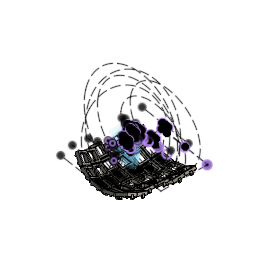
ArcBoard-mk6 v18 (Autodesk Fusion 360 design; units mm, degrees)
part number: mxledbit container
Autodesk Fusion 360 part; units mm, degrees
(part 1 of 5)
ref_plane "WorkPlane2" through (0, 16, 0) normal (0, 1, 0) x (0, 0, 1) in component "IND-Sketch"
sketch "IND-originXY" plane through (0, 0, 0) normal (0, 0, 1) x (1, 0, 0) in component "IND-Sketch"
  line L0 (0, 0) -> (0, 16) construction
  line L1 (0, 16) -> (16, 16) construction
  line L2 (16, 16) -> (16, 0) construction
  line L3 (16, 0) -> (0, 0) construction
  line L4 (0, 16) -> (8, 16) construction
  point P0 (8, 16)
  dimension "d20" = 16
  dimension "d21" = 16
  dimension "d29" = 16
  dimension "d30" = 16
  dimension "d34" = 8
  constraint coincident L0.start L3.end
  constraint vertical L0
  constraint perpendicular L0 L1
  constraint perpendicular L1 L2
  constraint perpendicular L0 L3
  constraint perpendicular L0 L4
  constraint coincident P0 L4.end
  measures "d20" distance of L0.start L0.end
  measures "d21" distance of L0.end L1.end
  measures "d29" distance of L1.end L2.end
  measures "d30" distance of L2.end L0.start
  measures "d34" distance of L0.end P0
sketch "IND-originXZ" plane through (0, 16, 0) normal (0, 1, 0) x (1, 0, 0) in component "IND-Sketch"
  line L0 (0, 0) -> (16, 0) construction
  line L1 (10, 0) -> (10, -10) construction
  line L2 (10, -10) -> (0, -10) construction
  line L3 (0, -10) -> (0, 0) construction
  line L4 (10, -10) -> (5, -10) construction
  line L5 (0, -10) -> (5, -10) construction
  line L6 (0, -10) -> (5, -10) construction
  point P0 (16, 0)
  point P1 (0, -10)
  point P2 (10, -10)
  point P3 (8, 0)
  point P4 (5, -10)
  dimension "d26" = 10
  dimension "d27" = 16
  dimension "d28" = 16
  dimension "d36" = 8
  dimension "d37" = 8
  constraint coincident P0 L1.start
  constraint perpendicular L0 L1
  constraint perpendicular L1 L2
  constraint coincident L0.start L3.end
  constraint coincident P1 L2.end
  constraint coincident P2 L1.end
  constraint midpoint L2 P4
  constraint perpendicular L1 L4
  constraint parallel L4 L6
  measures "d26" distance of L1.start P2
ref_plane "WorkPlane3" through (5, 16, 10) normal (0, 0.866025, -0.5) x (-1, 0, 0) in component "IND-Sketch"
sketch "IND-path" plane through (5, 15.25, 8.701) normal (0, 0.866025, -0.5) x (-1, 0, 0) in component "IND-Sketch"
  line L0 (-5, 1.5) -> (5, 1.5) construction
  line L1 (5, 1.5) -> (-5, 1.5) construction
  circle A0 centre (0, 0) radius 70 construction
  line L2 (0, 0) -> (8, 0) construction
  line L3 (0, 0) -> (-8, 0) construction
  line L4 (0, 0) -> (0, -70) construction
  line L5 (0, -70) -> (6.95, -70) construction
  line L6 (0, -70) -> (-6.95, -70) construction
  point P0 (-5, 1.5)
  point P1 (5, 1.5)
  point P2 (0, -70)
  dimension "d32" = 140
  dimension "d33" = 8
  dimension "d35" = 8
  dimension "d42" = 70
  dimension "d43" = 6.95
  dimension "d44" = 6.95
  dimension "d67" = 90
  constraint coincident P1 L0.end
  constraint coincident P0 L0.start
  constraint coincident A0.centre L2.start
  constraint parallel L1 L2
  constraint parallel L0 L3
  constraint coincident P2 L4.end
  constraint perpendicular L4 L5
  constraint perpendicular L4 L6
  measures "d32" diameter of A0
  measures "d33" distance of A0.centre L2.end
  measures "d35" distance of A0.centre L3.end
  measures "d42" distance of A0.centre P2
  measures "d43" distance of P2 L5.end
  measures "d44" distance of P2 L6.end
  measures "d67" angle of L2 L4
sketch "Sketch1" plane through (5, 15.25, 8.701) normal (0, 0.866025, -0.5) x (-1, 0, 0) in component "wheel"
  circle A0 centre (0, 0) radius 70
  line L0 (0, -70) -> (6.95, -70)
  line L1 (0, -70) -> (-6.95, -70)
  line L2 (0, -70) -> (0, 70) construction
  line L3 (0, 0) -> (70, 0) construction
  circle A1 centre (0, 0) radius 70
  point P0 (0, -70)
  point P1 (0, 1.5)
  dimension "d45" = 140
  dimension "d46" = 70
  dimension "d47" = 140
  constraint coincident P0 L0.start
  constraint perpendicular L0 L2
  constraint coincident A0.centre L3.start
  constraint perpendicular L2 L3
  measures "d45" distance of P0 L2.end
  measures "d46" distance of A0.centre L3.end
  measures "d47" diameter of A1
extrude "Extrude1" add sketch "Sketch1" along normal blind 4 makes body 1 in component "wheel"
ref_plane "WorkPlane1" through (5, -2.4532, -61.9071) normal (0, -0.5, -0.866025) x (1, 0, 0) in component "plug"
sketch "Sketch1 (2)" plane through (5, -4.7032, -60.6081) normal (0, -0.5, -0.866025) x (1, 0, 0) in component "plug"
  line L0 (-70, 13.3745) -> (70, 13.3745)
  line L1 (-70, 13.3745) -> (70, 13.3745)
  line L2 (-70, 17.3745) -> (70, 17.3745)
  line L3 (-70, 17.3745) -> (70, 17.3745)
  line L4 (0, 17.3745) -> (0, 13.3745) construction
  line L5 (0, 17.3745) -> (-6.95, 17.3745) construction
  line L6 (0, 17.3745) -> (6.95, 17.3745) construction
  line L7 (6.95, 17.3745) -> (6.95, 13.3745) construction
  line L8 (-6.95, 17.3745) -> (-6.95, 13.3745) construction
  line L9 (-6.95, 13.3745) -> (6.95, 13.3745) construction
  line L10 (6.95, 13.3745) -> (-6.95, 13.3745)
  line L11 (-6.95, 13.3745) -> (-6.95, 17.3745)
  line L12 (-6.95, 17.3745) -> (6.95, 17.3745)
  line L13 (6.95, 17.3745) -> (6.95, 13.3745)
  point P0 (0, 17.3745)
  dimension "d51" = 6.95
  dimension "d52" = 6.95
  constraint coincident P0 L4.start
  constraint midpoint L1 L4.end
  constraint perpendicular L4 L5
  constraint perpendicular L4 L6
  constraint coincident L1 L7.end
  constraint perpendicular L1 L7
  constraint coincident L0 L8.end
  constraint perpendicular L0 L8
  constraint horizontal L10
  constraint vertical L11
  constraint horizontal L12
  constraint vertical L13
  measures "d51" distance of P0 L5.end
  measures "d52" distance of P0 L6.end
extrude "Extrude1'" add sketch "Sketch1 (2)" along normal blind 4 separate body makes body 2 in component "plug"
sketch "Sketch2" plane through (0, -27.4199, -47.4926) normal (0, 0.5, 0.866025) x (1, 0, 0) in component "plug"
  line L0 (-1.95, 8.8564) -> (11.95, 8.8564)
  line L1 (11.95, 8.8564) -> (11.95, 12.8564)
  line L2 (11.95, 12.8564) -> (-1.95, 12.8564)
  line L3 (-1.95, 12.8564) -> (-1.95, 8.8564)
extrude "Extrude2" add 1 faces at (2.6833, -17.6192, -56.2302) along direction (0, 0.866025, -0.5) blind 4.95 on bodies 2 bodies 2 in component "plug"
extrude "Extrude3" add 1 faces at (7.3167, -20.4167, -53.0755) along direction (0, -0.866025, 0.5) blind 4.95 on bodies 2 bodies 2 in component "plug"
sketch "Sketch1 (3)" plane through (0, 0, 0) normal (0, 0, 1) x (1, 0, 0) in component "main-switchbody (1)"
  line L0 (0, 0) -> (0, 20) construction
  line L1 (0, 20) -> (20, 20) construction
  line L2 (20, 20) -> (20, 0) construction
  line L3 (20, 0) -> (0, 0) construction
  line L4 (0, 0) -> (20, 20) construction
  line L5 (20, 0) -> (0, 20) construction
  line L6 (10, 0) -> (18.9, 0) construction
  line L7 (10, 10) -> (18.9, 10) construction
  line L8 (18.9, 10) -> (18.9, 18.9) construction
  line L9 (18.9, 18.9) -> (1.1, 18.9) construction
  line L10 (1.1, 18.9) -> (1.1, 1.1) construction
  line L11 (1.1, 1.1) -> (18.9, 1.1) construction
  line L12 (18.9, 1.1) -> (18.9, 18.9) construction
  line L13 (10, 10) -> (3.05, 10) construction
  line L14 (3.05, 10) -> (3.05, 16.95) construction
  line L15 (3.05, 16.95) -> (16.95, 16.95) construction
  line L16 (16.95, 16.95) -> (16.95, 3.05) construction
  line L17 (16.95, 3.05) -> (3.05, 3.05) construction
  line L18 (3.05, 3.05) -> (3.05, 16.95) construction
  line L19 (3.05, 3.05) -> (0, 3.05) construction
  line L20 (3.05, 3.05) -> (3.05, 0) construction
  line L21 (16.95, 3.05) -> (20, 3.05) construction
  line L22 (16.95, 16.95) -> (20, 16.95) construction
  line L23 (16.95, 16.95) -> (16.95, 20) construction
  line L24 (3.05, 16.95) -> (3.05, 20) construction
  line L25 (3.05, 16.95) -> (0, 16.95) construction
  line L26 (3.05, 18.9) -> (6.05, 18.9) construction
  line L27 (6.05, 18.9) -> (6.05, 20) construction
  line L28 (16.95, 18.9) -> (13.95, 18.9) construction
  line L29 (13.95, 18.9) -> (13.95, 20) construction
  line L30 (16.95, 3.05) -> (16.95, 0) construction
  line L31 (16.95, 1.1) -> (13.95, 1.1) construction
  line L32 (13.95, 1.1) -> (13.95, 0) construction
  line L33 (3.05, 1.1) -> (6.05, 1.1) construction
  line L34 (6.05, 1.1) -> (6.05, 0) construction
  line L35 (0, 20) -> (20, 20) construction
  line L36 (20, 20) -> (20, 0) construction
  line L37 (20, 0) -> (0, 0) construction
  line L38 (0, 0) -> (0, 20) construction
  line L39 (0, 20) -> (20, 20)
  line L40 (20, 20) -> (20, 0)
  line L41 (20, 0) -> (0, 0)
  line L42 (0, 0) -> (0, 20)
  line L43 (16.95, 3.05) -> (3.05, 3.05)
  line L44 (3.05, 3.05) -> (3.05, 16.95)
  line L45 (3.05, 16.95) -> (16.95, 16.95)
  line L46 (16.95, 16.95) -> (16.95, 3.05)
  line L47 (3.05, 1.1) -> (6.05, 1.1)
  line L48 (6.05, 1.1) -> (6.05, 0)
  line L49 (6.05, 0) -> (3.05, 0)
  line L50 (3.05, 0) -> (3.05, 1.1)
  line L51 (13.95, 1.1) -> (16.95, 1.1)
  line L52 (16.95, 1.1) -> (16.95, 0)
  line L53 (16.95, 0) -> (13.95, 0)
  line L54 (13.95, 0) -> (13.95, 1.1)
  line L55 (13.95, 20) -> (16.95, 20)
  line L56 (16.95, 20) -> (16.95, 18.9)
  line L57 (16.95, 18.9) -> (13.95, 18.9)
  line L58 (13.95, 18.9) -> (13.95, 20)
  line L59 (3.05, 20) -> (6.05, 20)
  line L60 (6.05, 20) -> (6.05, 18.9)
  line L61 (6.05, 18.9) -> (3.05, 18.9)
  line L62 (3.05, 18.9) -> (3.05, 20)
  line L63 (1.1, 10) -> (1.1, 12)
  line L64 (1.1, 10) -> (1.1, 8)
  line L65 (1.1, 8) -> (-1.9, 8)
  line L66 (-1.9, 8) -> (1.1, 8)
  line L67 (1.1, 8) -> (1.1, 12)
  line L68 (1.1, 12) -> (-1.9, 12)
  line L69 (-1.9, 12) -> (-1.9, 8)
  line L70 (3.05, 10) -> (3.05, 7.5) construction
  line L71 (3.05, 7.5) -> (2.55, 7.5) construction
  line L72 (2.55, 7.5) -> (2.55, 12.5) construction
  line L73 (2.55, 12.5) -> (3.05, 12.5085) construction
  line L74 (3.05, 12.5085) -> (3.05, 7.5) construction
  line L75 (2.55, 12.5) -> (16.95, 12.5) construction
  line L76 (16.95, 12.5) -> (17.45, 12.5) construction
  line L77 (17.45, 12.5) -> (17.45, 7.5) construction
  line L78 (17.45, 7.5) -> (16.95, 7.5) construction
  line L79 (16.95, 7.5) -> (16.95, 12.5) construction
  line L80 (17.45, 7.5) -> (16.95, 7.5)
  line L81 (16.95, 7.5) -> (16.95, 12.5)
  line L82 (16.95, 12.5) -> (17.45, 12.5)
  line L83 (17.45, 12.5) -> (17.45, 7.5)
  line L84 (3.05, 7.5) -> (2.55, 7.5)
  line L85 (2.55, 7.5) -> (2.55, 12.5)
  line L86 (2.55, 12.5) -> (3.05, 12.5)
  line L87 (3.05, 12.5) -> (3.05, 7.5)
  dimension "d1_1" = 20
  dimension "d2_1" = 20
  dimension "d3_1" = 8.9
  dimension "d4_1" = 8.9
  dimension "d5_1" = 8.9
  dimension "d6_1" = 17.8
  dimension "d7_1" = 17.8
  dimension "d8_1" = 6.95
  dimension "d9_1" = 6.95
  dimension "d10_1" = 13.9
  dimension "d11_1" = 13.9
  dimension "d12_1" = 13.9
  dimension "d13_1" = 3
  dimension "d14_1" = 3
  dimension "d15_1" = 3
  dimension "d16_1" = 3
  dimension "d21_2" = 3
  dimension "d58_2" = 2.5
  dimension "d59_2" = 0.5
  dimension "d60_2" = 5
  dimension "d61_2" = 0.5
  dimension "d62_2" = 5
  constraint coincident L0.start L3.end
  constraint vertical L0
  constraint perpendicular L0 L1
  constraint perpendicular L1 L2
  constraint perpendicular L0 L3
  constraint midpoint L3 L6.start
  constraint parallel L3 L6
  constraint midpoint L4 L7.start
  constraint parallel L6 L7
  constraint perpendicular L7 L8
  constraint perpendicular L8 L9
  constraint perpendicular L9 L10
  constraint coincident L5 L11.end
  constraint perpendicular L10 L11
  constraint perpendicular L12 L13
  constraint perpendicular L13 L14
  constraint perpendicular L14 L15
  constraint perpendicular L7 L16
  constraint perpendicular L16 L17
  constraint coincident L0 L19.end
  constraint perpendicular L0 L19
  constraint coincident L3 L20.end
  constraint perpendicular L3 L20
  constraint coincident L2 L21.end
  constraint perpendicular L2 L21
  constraint coincident L2 L22.end
  constraint perpendicular L2 L22
  constraint coincident L1 L23.end
  constraint perpendicular L1 L23
  constraint coincident L1 L24.end
  constraint perpendicular L1 L24
  constraint coincident L0 L25.end
  constraint perpendicular L0 L25
  constraint coincident L24 L26.start
  constraint coincident L9 L26.start
  constraint coincident L9 L26.end
  constraint coincident L1 L27.end
  constraint perpendicular L1 L27
  constraint coincident L9 L28.start
  constraint coincident L23 L28.start
  constraint perpendicular L23 L28
  constraint coincident L1 L29.end
  constraint perpendicular L1 L29
  constraint coincident L6 L30.end
  constraint coincident L30 L31.start
  constraint coincident L11 L31.start
  constraint perpendicular L30 L31
  constraint coincident L6 L32.end
  constraint coincident L11 L33.start
  constraint coincident L20 L33.start
  constraint perpendicular L20 L33
  constraint coincident L3 L34.end
  constraint perpendicular L3 L34
  constraint horizontal L35
  constraint vertical L36
  constraint horizontal L37
  constraint vertical L38
  constraint horizontal L39
  constraint vertical L40
  constraint horizontal L41
  constraint vertical L42
  constraint horizontal L43
  constraint vertical L44
  constraint horizontal L45
  constraint vertical L46
  constraint horizontal L47
  constraint vertical L48
  constraint horizontal L49
  constraint vertical L50
  constraint horizontal L51
  constraint vertical L52
  constraint horizontal L53
  constraint vertical L54
  constraint horizontal L55
  constraint vertical L56
  constraint horizontal L57
  constraint vertical L58
  constraint horizontal L59
  constraint vertical L60
  constraint horizontal L61
  constraint vertical L62
  constraint midpoint L10 L63.start
  constraint coincident L10 L63.end
  constraint parallel L10 L63
  constraint coincident L10 L64.end
  constraint perpendicular L0 L65
  constraint horizontal L66
  constraint vertical L67
  constraint horizontal L68
  constraint vertical L69
  constraint perpendicular L13 L70
  constraint perpendicular L70 L71
  constraint perpendicular L71 L72
  constraint coincident L14 L73.end
  constraint perpendicular L71 L74
  constraint coincident L16 L75.end
  constraint perpendicular L16 L75
  constraint perpendicular L16 L76
  constraint perpendicular L76 L77
  constraint coincident L16 L78.end
  constraint perpendicular L16 L78
  constraint horizontal L80
  constraint vertical L81
  constraint horizontal L82
  constraint vertical L83
  constraint horizontal L84
  constraint vertical L85
  constraint horizontal L86
  constraint vertical L87
  measures "d1_1" distance of L0.start L0.end
  measures "d2_1" distance of L0.end L1.end
  measures "d3_1" distance of L6.start L6.end
  measures "d4_1" distance of L7.start L7.end
  measures "d5_1" distance of L7.end L8.end
  measures "d6_1" distance of L8.end L9.end
  measures "d7_1" distance of L9.end L10.end
  measures "d8_1" distance of L7.start L13.end
  measures "d9_1" distance of L13.end L14.end
  measures "d10_1" distance of L14.end L15.end
  measures "d11_1" distance of L15.end L16.end
  measures "d12_1" distance of L16.end L17.end
  measures "d13_1" distance of L26.start L26.end
  measures "d14_1" distance of L28.start L28.end
  measures "d15_1" distance of L31.start L31.end
  measures "d16_1" distance of L33.start L33.end
  measures "d21_2" distance of L64.end L65.end
  measures "d58_2" distance of L13.end L70.end
  measures "d59_2" distance of L70.end L71.end
  measures "d60_2" distance of L71.end L72.end
  measures "d61_2" distance of L75.end L76.end
  measures "d62_2" distance of L76.end L77.end
extrude "Extrude3'" add sketch "Sketch1 (3)" along normal blind 7.5 separate body contours L42 L63 L64 L65 L66 L67 L68 | L42 L65 L66 L68 L69 makes body 3 in component "main-switchbody (1)"
extrude "Extrude2'" add sketch "Sketch1 (3)" along normal blind 4 separate body contours L39 L40 L41 L42 L47 L48 L50 L51 L52 L54 L56 L57 L58 L60 L61 L62 L63 L64 L65 L66 L67 L68 | L42 L63 L64 L65 L66 L67 L68 | L46 L80 L81 L82 L83 | L44 L84 L85 L86 L87 makes body 4 in component "main-switchbody (1)"
extrude "Extrude1''" add sketch "Sketch1 (3)" along normal blind 6 separate body contours L39 L59 L60 L61 L62 | L39 L55 L56 L57 L58 | L41 L47 L48 L49 L50 | L41 L51 L52 L53 L54 makes body 5 at (4.05, 1.1, 2) makes body 6 at (5.05, 20, 4) makes body 7 at (14.95, 1.1, 2) makes body 8 at (14.95, 20, 2) in component "main-switchbody (1)"
extrude "Extrude4" cut sketch "Sketch1 (3)" along normal blind 2 contours L42 L65 L66 L68 L69 bodies 3 in component "main-switchbody (1)"
sketch "Sketch2 (2)" plane through (1.1, 0, 0) normal (1, 0, 0) x (0, 1, 0) in component "main-switchbody (1)"
  line L0 (8, 0) -> (12, 0)
  line L1 (12, 0) -> (12, 7.5)
  line L2 (12, 7.5) -> (8, 7.5)
  line L3 (8, 7.5) -> (8, 0)
  line L4 (8, 7.5) -> (8, 4) construction
  line L5 (8, 4) -> (12, 4) construction
  line L6 (12, 4) -> (12, 7.5) construction
  line L7 (12, 7.5) -> (8, 7.5) construction
  line L8 (8, 7.5) -> (8, 5.75) construction
  line L9 (8, 5.75) -> (12, 5.75) construction
  line L10 (8, 7.5) -> (12, 7.5)
  line L11 (12, 7.5) -> (12, 5.75)
  line L12 (12, 5.75) -> (8, 5.75)
  line L13 (8, 5.75) -> (8, 7.5)
  dimension "d26_2" = 1.75
  constraint coincident L2.end L3.start
  constraint coincident L3 L4.end
  constraint perpendicular L2 L4
  constraint coincident L1 L5.end
  constraint perpendicular L1 L5
  constraint coincident L1.end L2.start
  constraint perpendicular L2 L6
  constraint perpendicular L5 L8
  constraint midpoint L6 L9.end
  constraint horizontal L10
  constraint vertical L11
  constraint horizontal L12
  constraint vertical L13
  measures "d26_2" distance of L2.end L8.end
extrude "Extrude5" add sketch "Sketch2 (2)" along normal blind 1 contours L1 L2 L3 L10 L11 L12 L13 bodies 3 in component "main-switchbody (1)"
extrude "Extrude6" cut 1 faces at (-1.9, 10.6667, 3.8333) along direction (1, 0, 0) blind 1 on bodies 3 bodies 3 in component "main-switchbody (1)"
sketch "Sketch3" plane through (0, 18.9, 0) normal (0, -1, 0) x (1, 0, 0) in component "main-switchbody (1)"
  line L0 (3.05, 0) -> (6.05, 0)
  line L1 (6.05, 0) -> (6.05, 6)
  line L2 (6.05, 6) -> (3.05, 6)
  line L3 (3.05, 6) -> (3.05, 0)
  line L4 (3.05, 6) -> (3.05, 4) construction
  line L5 (6.05, 4) -> (6.05, 6) construction
  line L6 (3.05, 6) -> (3.05, 4.5) construction
  line L7 (6.05, 6) -> (6.05, 4.5) construction
  arc A0 (6.05, 4.5) -> (3.05, 4.5) centre (4.55, 4.5) ccw construction
  arc A1 (6.05, 4.5) -> (3.05, 4.5) centre (4.55, 4.5) ccw
  dimension "d31_2" = 1.5
  dimension "d32_2" = 1.5
  constraint coincident L2.end L3.start
  constraint coincident L3 L4.end
  constraint perpendicular L2 L4
  constraint coincident L1 L5.start
  constraint coincident L1.end L2.start
  constraint perpendicular L2 L5
  constraint perpendicular L2 L6
  constraint perpendicular L2 L7
  constraint tangent L2 A0
  constraint tangent L2 A1
  measures "d31_2" distance of L2.end L6.end
  measures "d32_2" distance of L1.end L7.end
extrude "Extrude7" cut sketch "Sketch3" against normal blind 1.1 contours L2 L3 A1 | L1 L2 A1 bodies 6 in component "main-switchbody (1)"
sketch "Sketch4" plane through (0, 0, 0) normal (0, -1, 0) x (1, 0, 0) in component "main-switchbody (1)"
  line L0 (3.05, 0) -> (6.05, 0)
  line L1 (6.05, 0) -> (6.05, 6)
  line L2 (6.05, 6) -> (3.05, 6)
  line L3 (3.05, 6) -> (3.05, 0)
  line L4 (3.05, 6) -> (3.05, 4.5) construction
  line L5 (6.05, 6) -> (6.05, 4.5) construction
  arc A0 (6.05, 4.5) -> (3.05, 4.5) centre (4.55, 4.5) ccw
  constraint coincident L2.end L3.start
  constraint coincident L3 L4.end
  constraint perpendicular L2 L4
  constraint coincident L1.end L2.start
  constraint coincident L1 L5.end
  constraint perpendicular L2 L5
  constraint tangent L2 A0
extrude "Extrude8" cut sketch "Sketch4" against normal blind 1.1 contours L2 L3 A0 | L1 L2 A0 bodies 5 in component "main-switchbody (1)"
sketch "Sketch5" plane through (0, 0, 0) normal (0, -1, 0) x (1, 0, 0) in component "main-switchbody (1)"
  line L0 (13.95, 0) -> (16.95, 0)
  line L1 (16.95, 0) -> (16.95, 6)
  line L2 (16.95, 6) -> (13.95, 6)
  line L3 (13.95, 6) -> (13.95, 0)
  line L4 (13.95, 6) -> (13.95, 4.5) construction
  line L5 (16.95, 6) -> (16.95, 4.5) construction
  arc A0 (16.95, 4.5) -> (13.95, 4.5) centre (15.45, 4.5) ccw
  constraint coincident L2.end L3.start
  constraint coincident L3 L4.end
  constraint perpendicular L2 L4
  constraint coincident L1.end L2.start
  constraint coincident L1 L5.end
  constraint perpendicular L2 L5
  constraint tangent L2 A0
extrude "Extrude9" cut sketch "Sketch5" against normal blind 1.1 contours L2 L3 A0 | L1 L2 A0 bodies 7 in component "main-switchbody (1)"
sketch "Sketch6" plane through (0, 18.9, 0) normal (0, -1, 0) x (1, 0, 0) in component "main-switchbody (1)"
  line L0 (13.95, 0) -> (16.95, 0)
  line L1 (16.95, 0) -> (16.95, 6)
  line L2 (16.95, 6) -> (13.95, 6)
  line L3 (13.95, 6) -> (13.95, 0)
  line L4 (13.95, 6) -> (13.95, 4.5) construction
  line L5 (16.95, 6) -> (16.95, 4.5) construction
  arc A0 (16.95, 4.5) -> (13.95, 4.5) centre (15.45, 4.5) ccw
  constraint coincident L2.end L3.start
  constraint coincident L3 L4.end
  constraint perpendicular L2 L4
  constraint coincident L1.end L2.start
  constraint coincident L1 L5.end
  constraint perpendicular L2 L5
  constraint tangent L2 A0
extrude "Extrude10" cut sketch "Sketch6" against normal blind 1.1 contours L2 L3 A0 | L1 L2 A0 bodies 8 in component "main-switchbody (1)"
sketch "Sketch7" plane through (0, 0, 4) normal (0, 0, 1) x (-1, 0, 0) in component "main-switchbody (1)"
  line L0 (-3.05, -16.95) -> (-16.95, -16.95)
  line L1 (-16.95, -16.95) -> (-16.95, -3.05)
  line L2 (-16.95, -3.05) -> (-3.05, -3.05)
  line L3 (-3.05, -3.05) -> (-3.05, -16.95)
  line L4 (-6.05, -20) -> (-6.05, -18.9)
  line L5 (-6.05, -18.9) -> (-3.05, -18.9)
  line L6 (-3.05, -18.9) -> (-3.05, -20)
  line L7 (-3.05, -20) -> (0, -20)
  line L8 (0, -20) -> (0, 0)
  line L9 (0, 0) -> (-3.05, 0)
  line L10 (-3.05, 0) -> (-3.05, -1.1)
  line L11 (-3.05, -1.1) -> (-6.05, -1.1)
  line L12 (-6.05, -1.1) -> (-6.05, 0)
  line L13 (-6.05, 0) -> (-13.95, 0)
  line L14 (-13.95, 0) -> (-13.95, -1.1)
  line L15 (-13.95, -1.1) -> (-16.95, -1.1)
  line L16 (-16.95, -1.1) -> (-16.95, 0)
  line L17 (-16.95, 0) -> (-20, 0)
  line L18 (-20, 0) -> (-20, -20)
  line L19 (-20, -20) -> (-16.95, -20)
  line L20 (-16.95, -20) -> (-16.95, -18.9)
  line L21 (-16.95, -18.9) -> (-13.95, -18.9)
  line L22 (-13.95, -18.9) -> (-13.95, -20)
  line L23 (-13.95, -20) -> (-6.05, -20)
  line L24 (-20, -10) -> (-20, -11.5) construction
  line L25 (-20, -10) -> (-20, -8.5) construction
  line L26 (-20, -8.5) -> (-19, -8.5) construction
  line L27 (-19, -8.5) -> (-19, -11.5) construction
  line L28 (-19, -11.5) -> (-20, -11.5) construction
  line L29 (-20, -11.5) -> (-21, -11.5) construction
  line L30 (-21, -11.5) -> (-21, -8.5) construction
  line L31 (-21, -8.5) -> (-20, -8.5) construction
  line L32 (-19, -11.5) -> (-21, -11.5)
  line L33 (-21, -11.5) -> (-21, -8.5)
  line L34 (-21, -8.5) -> (-19, -8.5)
  line L35 (-19, -8.5) -> (-19, -11.5)
  dimension "d41_2" = 1.5
  dimension "d42_2" = 1
  constraint midpoint L18 L24.start
  constraint parallel L18 L24
  constraint coincident L18 L25.end
  constraint parallel L18 L25
  constraint perpendicular L25 L26
  constraint perpendicular L26 L27
  constraint perpendicular L24 L29
  constraint perpendicular L29 L30
  constraint horizontal L32
  constraint vertical L33
  constraint horizontal L34
  constraint vertical L35
  measures "d41_2" distance of L24.start L24.end
  measures "d42_2" distance of L24.end L29.end
extrude "Extrude11" add sketch "Sketch7" along normal blind 3 contours L18 L32 L33 L34 | L18 L32 L34 L35 bodies 4 in component "main-switchbody (1)"
extrude "Extrude12" add 1 faces at (20, 8.5, 6) along direction (0, -1, 0) blind 0.5 on bodies 4 bodies 4 in component "main-switchbody (1)"
extrude "Extrude13" add 1 faces at (20, 11.5, 6) along direction (0, 1, 0) blind 0.5 on bodies 4 bodies 4 in component "main-switchbody (1)"
extrude "Extrude14" add 1 faces at (20.3333, 10.6667, 7) along direction (0, 0, 1) blind 0.75 on bodies 4 bodies 4 in component "main-switchbody (1)"
sketch "Sketch8" plane through (0, 0, 4) normal (0, 0, -1) x (1, 0, 0) in component "main-switchbody (1)"
  line L0 (20, -8) -> (20, -12)
  line L1 (20, -12) -> (21, -12)
  line L2 (21, -12) -> (21, -8)
  line L3 (21, -8) -> (20, -8)
  line L4 (20, -12) -> (20, -8)
  constraint coincident L0.end L1.start
  constraint coincident L0.start L3.end
extrude "Extrude15" add sketch "Sketch8" along normal blind 2 bodies 4 in component "main-switchbody (1)"
sketch "Sketch9" plane through (19, 0, 0) normal (-1, 0, 0) x (0, -1, 0) in component "main-switchbody (1)"
  line L0 (-12, 4) -> (-8, 4)
  line L1 (-8, 4) -> (-8, 7.75)
  line L2 (-8, 7.75) -> (-12, 7.75)
  line L3 (-12, 7.75) -> (-12, 4)
  line L4 (-12, 7.75) -> (-12, 5.75) construction
  line L5 (-12, 5.75) -> (-8, 5.75) construction
  line L6 (-12, 7.75) -> (-8, 7.75)
  line L7 (-8, 7.75) -> (-8, 5.75)
  line L8 (-8, 5.75) -> (-12, 5.75)
  line L9 (-12, 5.75) -> (-12, 7.75)
  dimension "d53_2" = 2
  constraint coincident L2.end L3.start
  constraint perpendicular L2 L4
  constraint coincident L1 L5.end
  constraint perpendicular L1 L5
  constraint horizontal L6
  constraint vertical L7
  constraint horizontal L8
  constraint vertical L9
  measures "d53_2" distance of L2.end L4.end
extrude "Extrude16" add sketch "Sketch9" along normal blind 0.5 contours L1 L2 L3 L6 L7 L8 L9 bodies 4 in component "main-switchbody (1)"
extrude "Extrude17" cut 1 faces at (2.1, 9.3333, 6.9167) along direction (-1, 0, 0) blind 0.3 on bodies 3 bodies 3 in component "main-switchbody (1)"
extrude "Extrude18" cut sketch "Sketch1 (3)" along normal blind 2.7 contours L44 L84 L85 L86 L87 bodies 4 in component "main-switchbody (1)"
extrude "Extrude19" cut sketch "Sketch1 (3)" along normal blind 2.7 contours L46 L80 L81 L82 L83 bodies 4 in component "main-switchbody (1)"
extrude "Extrude20" add sketch "Sketch1 (3)" against normal blind 0.2 contours L39 L40 L41 L42 L47 L48 L50 L51 L52 L54 L56 L57 L58 L60 L61 L62 L63 L64 L65 L66 L67 L68 | L39 L59 L60 L61 L62 | L42 L63 L64 L65 L66 L67 L68 | L39 L55 L56 L57 L58 | L41 L47 L48 L49 L50 | L41 L51 L52 L53 L54 bodies 3 4 5 6 7 8 in component "main-switchbody (1)"
fillet "Fillet1" radius 1 2 edges at (21, 10, 7.75) (-0.9, 10, 7.5) on bodies 3 4 in component "main-switchbody (1)"
extrude "Extrude21" add 1 faces at (2.8833, 9.1667, 2.7) along direction (0, 0, -1) blind 2.9 on bodies 3 bodies 3 in component "main-switchbody (1)"
extrude "Extrude22" add 1 faces at (17.1167, 10.8333, 2.7) along direction (0, 0, -1) blind 2.9 on bodies 3 bodies 3 in component "main-switchbody (1)"
sketch "Sketch10" plane through (0, 0, 4) normal (0, 0, 1) x (-1, 0, 0) in component "main-switchbody (1)"
  line L0 (-3.05, -16.95) -> (-16.95, -16.95)
  line L1 (-16.95, -16.95) -> (-16.95, -3.05)
  line L2 (-16.95, -3.05) -> (-3.05, -3.05)
  line L3 (-3.05, -3.05) -> (-3.05, -16.95)
  line L4 (0, -12) -> (-1.1, -12)
  line L5 (-1.1, -12) -> (-1.1, -8)
  line L6 (-1.1, -8) -> (0, -8)
  line L7 (0, -8) -> (0, 0)
  line L8 (0, 0) -> (-3.05, 0)
  line L9 (-3.05, 0) -> (-3.05, -1.1)
  line L10 (-3.05, -1.1) -> (-6.05, -1.1)
  line L11 (-6.05, -1.1) -> (-6.05, 0)
  line L12 (-6.05, 0) -> (-13.95, 0)
  line L13 (-13.95, 0) -> (-13.95, -1.1)
  line L14 (-13.95, -1.1) -> (-16.95, -1.1)
  line L15 (-16.95, -1.1) -> (-16.95, 0)
  line L16 (-16.95, 0) -> (-20, 0)
  line L17 (-20, 0) -> (-20, -8)
  line L18 (-20, -8) -> (-19, -8)
  line L19 (-19, -8) -> (-19, -12)
  line L20 (-19, -12) -> (-20, -12)
  line L21 (-20, -12) -> (-20, -20)
  line L22 (-20, -20) -> (-16.95, -20)
  line L23 (-16.95, -20) -> (-16.95, -18.9)
  line L24 (-16.95, -18.9) -> (-13.95, -18.9)
  line L25 (-13.95, -18.9) -> (-13.95, -20)
  line L26 (-13.95, -20) -> (-6.05, -20)
  line L27 (-6.05, -20) -> (-6.05, -18.9)
  line L28 (-6.05, -18.9) -> (-3.05, -18.9)
  line L29 (-3.05, -18.9) -> (-3.05, -20)
  line L30 (-3.05, -20) -> (0, -20)
  line L31 (0, -20) -> (0, -12)
  line L32 (-3.05, -10) -> (-3.05, -12.5) construction
  line L33 (-3.05, -12.5) -> (-3.05, -7.5) construction
  line L34 (-3.05, -7.5) -> (-2.55, -7.5) construction
  line L35 (-2.55, -7.5) -> (-3.05, -7.5) construction
  line L36 (-3.05, -7.5) -> (-3.05, -12.5) construction
  line L37 (-3.05, -12.5) -> (-2.55, -12.5) construction
  line L38 (-2.55, -12.5) -> (-2.55, -7.5) construction
  line L39 (-3.05, -12.5) -> (-16.95, -12.5) construction
  line L40 (-16.95, -12.5) -> (-16.95, -7.5) construction
  line L41 (-16.95, -7.5) -> (-17.45, -7.5) construction
  line L42 (-17.45, -7.5) -> (-16.95, -7.5) construction
  line L43 (-16.95, -7.5) -> (-16.95, -12.5) construction
  line L44 (-16.95, -12.5) -> (-17.45, -12.5) construction
  line L45 (-17.45, -12.5) -> (-17.45, -7.5) construction
  line L46 (-16.95, -12.5) -> (-17.45, -12.5)
  line L47 (-17.45, -12.5) -> (-17.45, -7.5)
  line L48 (-17.45, -7.5) -> (-16.95, -7.5)
  line L49 (-16.95, -7.5) -> (-16.95, -12.5)
  line L50 (-2.55, -12.5) -> (-3.05, -12.5)
  line L51 (-3.05, -12.5) -> (-3.05, -7.5)
  line L52 (-3.05, -7.5) -> (-2.55, -7.5)
  line L53 (-2.55, -7.5) -> (-2.55, -12.5)
  dimension "d75_1" = 5
  dimension "d76_1" = 0.5
  dimension "d77_1" = 0.5
  constraint midpoint L3 L32.start
  constraint coincident L3 L32.end
  constraint perpendicular L0 L32
  constraint parallel L3 L33
  constraint perpendicular L33 L34
  constraint horizontal L35
  constraint vertical L36
  constraint horizontal L37
  constraint vertical L38
  constraint coincident L1 L39.end
  constraint perpendicular L1 L39
  constraint coincident L1 L40.end
  constraint perpendicular L39 L40
  constraint perpendicular L40 L41
  constraint horizontal L42
  constraint vertical L43
  constraint horizontal L44
  constraint vertical L45
  constraint horizontal L46
  constraint vertical L47
  constraint horizontal L48
  constraint vertical L49
  constraint horizontal L50
  constraint vertical L51
  constraint horizontal L52
  constraint vertical L53
  measures "d75_1" distance of L32.end L33.end
  measures "d76_1" distance of L33.end L34.end
  measures "d77_1" distance of L40.end L41.end
extrude "Extrude23" cut sketch "Sketch10" against normal blind 2.9 contours L3 L50 L51 L52 L53 | L1 L46 L47 L48 L49 bodies 3 in component "main-switchbody (1)"
extrude "Extrude24" cut 2 faces at (4.8122, 18.9, 5.1079) (15.1626, 18.9, 5.4316) along direction (0, 1, 0) blind 0.25 on bodies 3 bodies 3 in component "main-switchbody (1)"
extrude "Extrude25" cut 2 faces at (4.2822, 1.1, 5.1824) (15.2673, 1.1, 4.9654) along direction (0, -1, 0) blind 0.25 on bodies 3 bodies 3 in component "main-switchbody (1)"
extrude "Extrude26" add 1 faces at (1.0167, 12.3167, -0.2) along direction (0, 0, -1) blind 1 on bodies 3 bodies 3 in component "main-switchbody (1)"
extrude "Extrude27" cut 1 faces at (1.0167, 12.3167, -1.2) along direction (0, 0, 1) blind 0.2 on bodies 3 bodies 3 in component "main-switchbody (1)"
extrude "Extrude28" cut 2 faces at (17.1167, 10.8333, 1.1) (2.8833, 9.1667, 1.1) along direction (0, 0, -1) blind 0.8 on bodies 3 bodies 3 in component "main-switchbody (1)"
extrude "Extrude29" cut 1 faces at (18.8333, 9.3333, 5.75) along direction (0, 0, 1) blind 0.2 on bodies 3 bodies 3 in component "main-switchbody (1)"
extrude "Extrude30" cut 1 faces at (1.3333, 10.6667, 5.75) along direction (0, 0, 1) blind 0.2 on bodies 3 bodies 3 in component "main-switchbody (1)"
sketch "Sketch1 (4)" plane through (0, 0, 0.0152) normal (0, 0, -1) x (1, 0, 0) in component "mxledbit-switchbody v10 (1)"
  line L0 (4.5419, -16.2374) -> (4.5419, -2.3374)
  line L1 (4.5419, -2.3374) -> (18.4419, -2.3374)
  line L2 (18.4419, -2.3374) -> (18.4419, -16.2374)
  line L3 (18.4419, -16.2374) -> (4.5419, -16.2374)
  line L4 (1.4919, -19.2874) -> (21.4919, -19.2874)
  line L5 (21.4919, -19.2874) -> (21.4919, 0.7126)
  line L6 (21.4919, 0.7126) -> (1.4919, 0.7126)
  line L7 (1.4919, 0.7126) -> (1.4919, -19.2874)
ref_plane "WorkPlane1" through (5, 16.9821, 7.701) normal (0, -0.866025, 0.5) x (1, 0, 0) in component "wheel"
sketch "Sketch2 (3)" plane through (5, 16.9821, 7.701) normal (0, -0.866025, 0.5) x (1, 0, 0) in component "wheel"
  circle A0 centre (0, 0) radius 70
  dimension "d64" = 140
  constraint coincident A0.centre origin
  measures "d64" diameter of A0
component_pattern "component pattern" in component "Index1"
sketch "Sketch2 (4)" plane through (0, 7.6699, -4.4282) normal (0, -0.866025, 0.5) x (1, 0, 0) in component "IND-Sketch"
  circle A0 centre (5, 15.1603) radius 70
  line L0 (5, 15.1603) -> (5, -54.8397) construction
  line L1 (5, -54.8397) -> (-3, -54.8397) construction
  line L2 (-3, -54.8397) -> (13, -54.8397)
  line L3 (13, -54.8397) -> (13, 15.1603)
  line L4 (13, 15.1603) -> (-3, 15.1603)
  line L5 (-3, 15.1603) -> (-3, -54.8397)
  dimension "d69" = 70
  dimension "d70" = 8
  dimension "d71" = 16
  dimension "d72" = 70
  constraint coincident A0.centre L0.start
  constraint vertical L0
  constraint perpendicular L0 L1
  constraint horizontal L2
  constraint vertical L3
  constraint horizontal L4
  constraint vertical L5
  measures "d69" distance of A0.centre L0.end
  measures "d70" distance of L0.end L1.end
  measures "d71" distance of L1.end L2.end
  measures "d72" distance of L1.end L4.end
sketch "Sketch9 (2)" plane through (5, 41.9534, 55.6343) normal (0, 0.573576, 0.819152) x (-1, 0, 0) in component "IND-Sketch"
  line L0 (-45, -9.823) -> (5, -9.823) construction
  line L1 (-20, -9.823) -> (5, -9.823) construction
  line L2 (-20, -9.823) -> (-45, -9.823) construction
  circle A0 centre (-20, -9.823) radius 75 construction
  point P0 (-20, -9.823)
  point P1 (-45, -9.823)
  point P2 (5, -9.823)
  point P3 (5, -9.823)
  point P4 (-45, -9.823)
  dimension "d38" = 16
  dimension "d39" = 8
  dimension "d40" = 8
  dimension "d41" = 140
  constraint coincident P4 P1
  constraint horizontal L0
  constraint coincident P0 L1.start
  constraint parallel L0 L1
  constraint parallel L0 L2
sketch "Sketch1 (5)" plane through (0, 54.7581, -45.9475) normal (0, -0.766044, 0.642788) x (1, 0, 0) in component "IND-Sketch"
  line L0 (-1.3269, 70.632) -> (-1.3269, 84.532)
  line L1 (-1.3269, 84.532) -> (12.5731, 84.532)
  line L2 (12.5731, 84.532) -> (12.5731, 70.632)
  line L3 (12.5731, 70.632) -> (-1.3269, 70.632)
  line L4 (-4.3769, 67.582) -> (15.6231, 67.582)
  line L5 (15.6231, 67.582) -> (15.6231, 87.582)
  line L6 (15.6231, 87.582) -> (-4.3769, 87.582)
  line L7 (-4.3769, 87.582) -> (-4.3769, 67.582)
  line L8 (-4.3769, 77.582) -> (15.6231, 77.582) construction
  line L9 (5.6231, 87.582) -> (5.6231, 67.582) construction
  point P0 (5.6231, 77.582)
  constraint midpoint L7 L8.start
  constraint midpoint L5 L8.end
  constraint midpoint L6 L9.start
  constraint midpoint L4 L9.end
  constraint midpoint L8 P0
  measures "d69" distance of L9.end
  measures "d70" distance of L9.end
  measures "d69_1" distance of L9.end
  measures "d70_1" distance of L9.end
  measures "d69_3" distance of L9.end
  measures "d70_3" distance of L9.end
  measures "d69_7" distance of L9.end
  measures "d70_7" distance of L9.end
  measures "d69_10" distance of L9.end
  measures "d70_10" distance of L9.end
  measures "d69_13" distance of L9.end
  measures "d70_13" distance of L9.end
ref_plane "WorkPlane2" through (0, 30, 0) normal (0, 1, 0) x (0, 0, 1) in component "IND-Sketch (1)"
sketch "IND-originXY (2)" plane through (0, 0, 0) normal (0, 0, 1) x (1, 0, 0) in component "IND-Sketch (1)"
  line L0 (0, 0) -> (0, 16) construction
  line L1 (0, 16) -> (16, 16) construction
  line L2 (16, 16) -> (16, -14) construction
  line L3 (16, -14) -> (-14, -14) construction
  line L4 (0, 16) -> (15, 16) construction
  point P0 (15, 16)
  dimension "d20_1" = 16
  dimension "d21_1" = 16
  dimension "d29_1" = 30
  dimension "d30_1" = 30
  dimension "d34_1" = 15
  constraint coincident L0.start origin
  constraint vertical L0
  constraint perpendicular L0 L1
  constraint perpendicular L1 L2
  constraint perpendicular L0 L3
  constraint perpendicular L0 L4
  constraint coincident P0 L4.end
  measures "d20_1" distance of L0.start L0.end
  measures "d21_1" distance of L0.end L1.end
  measures "d29_1" distance of L1.end L2.end
  measures "d30_1" distance of L2.end L3.end
  measures "d34_1" distance of L0.end P0
sketch "IND-originXZ (2)" plane through (0, 30, 0) normal (0, 1, 0) x (1, 0, 0) in component "IND-Sketch (1)"
  line L0 (0, 0) -> (16, 0) construction
  line L1 (10, 0) -> (10, -10) construction
  line L2 (10, -10) -> (0, -10) construction
  line L3 (0, -10) -> (0, 0) construction
  line L4 (10, -10) -> (5, -10) construction
  line L5 (0, -10) -> (5, -10) construction
  line L6 (0, -10) -> (5, -10) construction
  point P0 (16, 0)
  point P1 (0, -10)
  point P2 (10, -10)
  point P3 (15, 0)
  point P4 (5, -10)
  dimension "d26_1" = 0
  dimension "d27_1" = 30
  dimension "d28_1" = 30
  dimension "d36_1" = 15
  dimension "d37_1" = 15
  constraint coincident P0 L1.start
  constraint perpendicular L0 L1
  constraint perpendicular L1 L2
  constraint coincident L0.start L3.end
  constraint coincident P1 L2.end
  constraint coincident P2 L1.end
  constraint midpoint L2 P4
  constraint perpendicular L1 L4
  constraint parallel L4 L6
  measures "d26_1" distance of L1.start P2
ref_plane "WorkPlane3" through (5, 30, 10) normal (0, 0.939693, -0.34202) x (-1, 0, 0) in component "IND-Sketch (1)"
sketch "IND-path (2)" plane through (5, 30, 10) normal (0, 0.939693, -0.34202) x (-1, 0, 0) in component "IND-Sketch (1)"
  line L0 (-5, 0) -> (5, 0) construction
  line L1 (5, 0) -> (-5, 0) construction
  circle A0 centre (0, 0) radius 80 construction
  line L2 (0, 0) -> (15, 0) construction
  line L3 (0, 0) -> (-15, 0) construction
  line L4 (0, 0) -> (0, -80) construction
  line L5 (0, -80) -> (6.95, -80) construction
  line L6 (0, -80) -> (-6.95, -80) construction
  point P0 (-5, 0)
  point P1 (5, 0)
  point P2 (0, -80)
  dimension "d32_1" = 160
  dimension "d33_1" = 15
  dimension "d35_1" = 15
  dimension "d42_1" = 80
  dimension "d43_1" = 6.95
  dimension "d44_1" = 6.95
  dimension "d67_1" = 90
  constraint coincident P1 L0.end
  constraint coincident P0 L0.start
  constraint coincident A0.centre L2.start
  constraint parallel L1 L2
  constraint parallel L0 L3
  constraint coincident P2 L4.end
  constraint perpendicular L4 L5
  constraint perpendicular L4 L6
  measures "d32_1" diameter of A0
  measures "d33_1" distance of A0.centre L2.end
  measures "d35_1" distance of A0.centre L3.end
  measures "d42_1" distance of A0.centre P2
  measures "d43_1" distance of P2 L5.end
  measures "d44_1" distance of P2 L6.end
  measures "d67_1" angle of L2 L4
sketch "Sketch1 (6)" plane through (5, 30, 10) normal (0, 0.939693, -0.34202) x (-1, 0, 0) in component "wheel (1)"
  circle A0 centre (0, 0) radius 80
  line L0 (0, -80) -> (6.95, -80)
  line L1 (0, -80) -> (-6.95, -80)
  line L2 (0, -80) -> (0, 80) construction
  line L3 (0, 0) -> (80, 0) construction
  circle A1 centre (0, 0) radius 80
  point P0 (0, -80)
  dimension "d45_1" = 160
  dimension "d46_1" = 80
  dimension "d47_1" = 160
  constraint coincident P0 L0.start
  constraint perpendicular L0 L2
  constraint coincident A0.centre L3.start
  constraint perpendicular L2 L3
  measures "d45_1" distance of P0 L2.end
  measures "d46_1" distance of A0.centre L3.end
  measures "d47_1" diameter of A1
extrude "Extrude1'''" add sketch "Sketch1 (6)" along normal blind 4 separate body makes body 9 in component "wheel (1)"
ref_plane "WorkPlane1" through (5, 24.0876, -72.9823) normal (0, -0.34202, -0.939693) x (1, 0, 0) in component "plug (1)"
sketch "Sketch1 (7)" plane through (5, 22.747, -72.4944) normal (0, -0.34202, -0.939693) x (1, 0, 0) in component "plug (1)"
  line L0 (-80, 17.3992) -> (80, 17.3992)
  line L1 (-80, 17.3992) -> (80, 17.3992)
  line L2 (-80, 21.3992) -> (80, 21.3992)
  line L3 (-80, 21.3992) -> (80, 21.3992)
  line L4 (0, 21.3992) -> (0, 17.3992) construction
  line L5 (0, 21.3992) -> (-6.95, 21.3992) construction
  line L6 (0, 21.3992) -> (6.95, 21.3992) construction
  line L7 (6.95, 21.3992) -> (6.95, 17.3992) construction
  line L8 (-6.95, 21.3992) -> (-6.95, 17.3992) construction
  line L9 (-6.95, 17.3992) -> (6.95, 17.3992) construction
  line L10 (6.95, 17.3992) -> (-6.95, 17.3992)
  line L11 (-6.95, 17.3992) -> (-6.95, 21.3992)
  line L12 (-6.95, 21.3992) -> (6.95, 21.3992)
  line L13 (6.95, 21.3992) -> (6.95, 17.3992)
  point P0 (0, 21.3992)
  dimension "d51_1" = 6.95
  dimension "d52_1" = 6.95
  constraint coincident P0 L4.start
  constraint midpoint L1 L4.end
  constraint perpendicular L4 L5
  constraint perpendicular L4 L6
  constraint coincident L1 L7.end
  constraint perpendicular L1 L7
  constraint coincident L0 L8.end
  constraint perpendicular L0 L8
  constraint horizontal L10
  constraint vertical L11
  constraint horizontal L12
  constraint vertical L13
  measures "d51_1" distance of P0 L5.end
  measures "d52_1" distance of P0 L6.end
extrude "Extrude1''''" add sketch "Sketch1 (7)" along normal blind 4 separate body makes body 10 in component "plug (1)"
sketch "Sketch2 (5)" plane through (0, -20.6383, -56.7034) normal (0, 0.34202, 0.939693) x (1, 0, 0) in component "plug (1)"
  line L0 (-1.95, 24.7706) -> (11.95, 24.7706)
  line L1 (11.95, 24.7706) -> (11.95, 28.7706)
  line L2 (11.95, 28.7706) -> (-1.95, 28.7706)
  line L3 (-1.95, 28.7706) -> (-1.95, 24.7706)
extrude "Extrude2''" add 1 faces at (7.3167, 5.9411, -67.7964) along direction (0, 0.939693, -0.34202) blind 4.95 on bodies 10 bodies 10 in component "plug (1)"
extrude "Extrude3''" add 1 faces at (2.6833, 1.7263, -67.6813) along direction (0, -0.939693, 0.34202) blind 4.95 on bodies 10 bodies 10 in component "plug (1)"